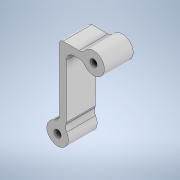
# Autodesk Inventor part: back
Saved by Autodesk Inventor 2021 (Build 250183000, 183)
## iProperties
Created: 2025-12-28
Part Number: back
Material: Generic
Document SubType Name: Modeling
Designer: Toby
Density: 1 g/cm^3
Appearance: Default
Author: Toby
Autodesk Inventor part; units mm, degrees
ref_plane "YZ Plane" through (0, 0, 0) normal (1, 0, 0) x (0, 1, 0)
ref_plane "XZ Plane" through (0, 0, 0) normal (0, 1, 0) x (-1, 0, 0)
ref_plane "XY Plane" through (0, 0, 0) normal (0, 0, 1) x (1, 0, 0)
sketch "Sketch1" plane through (0, 0, 0) normal (0, 0, 1) x (1, 0, 0)
  circle A0 centre (-5, -11) radius 3
  circle A1 centre (5, 11) radius 3
  point P0 (0, 0)
  dimension "d0" = 10
  dimension "d1" = 22
  dimension "d2" = 5
  dimension "d3" = 11
  dimension "d4" = 6
  dimension "d5" = 6
  constraints: 2 centre point, 2 coincident
  measures "d0" horizontal distance of point (-5, -11) point (5, 11)
  measures "d1" vertical distance of point (-5, -11) point (5, 11)
  measures "d2" horizontal distance of point (0, 0) point (-5, -11)
  measures "d3" vertical distance of point (-5, -11) point (0, 0)
  measures "d4" diameter of A0
  measures "d5" diameter of A1
extrude "Extrusion1" add sketch "Sketch1" along normal blind 8
sketch "Sketch2" plane through (5, 11, 8) normal (0, 0, 1) x (1, 0, 0)
  circle A0 centre (0, 0) radius 3 projected
  circle A1 centre (-10, -22) radius 3 projected
  line L0 (-10, -22) -> (-8.5, -18) construction
  line L1 (-9.0637, -22.3511) -> (-7.5637, -18.3511)
  line L2 (-9.4363, -17.6489) -> (-10.9363, -21.6489)
  arc A2 (-10.9363, -21.6489) -> (-9.0637, -22.3511) centre (-10, -22) ccw
  arc A3 (-7.5637, -18.3511) -> (-9.4363, -17.6489) centre (-8.5, -18) ccw
  circle A4 centre (-8.5, 0) radius 1
  point P0 (-5, -11)
  point P1 (-10, -19)
  point P2 (-9.25, -20)
  dimension "d8" = 0
  dimension "d9" = 1.5
  dimension "d10" = 3
  dimension "d11" = 0
  dimension "d12" = 1.5
  dimension "d13" = 4
  dimension "d14" = 2
  dimension "d15" = 2
  constraints: 8 end point, 4 point on circle, 4 tangent, 3 centre point, 1 coincident, 1 midpoint, 1 parallel
  measures "d8" vertical distance of A0.centre point (-8.5, 0)
  measures "d9" horizontal distance of L0.start point (-8.5, 0)
  measures "d10" distance of L0.start point (-10, -19)
  measures "d11" horizontal distance of L0.start point (-10, -19)
  measures "d12" horizontal distance of L0.start L0.end
  measures "d13" vertical distance of L0.start L0.end
  measures "d14" diameter of A3
  measures "d15" diameter of A4
extrude "Extrusion2" add sketch "Sketch2" against normal blind 8 contours L1 A2 L2 A1 | A1 L2 A3 L1 | A4 picked at (-9.757, -21.03)
sketch "Sketch3" plane through (-3.5, 11, 8) normal (0, 0, 1) x (1, 0, 0)
  circle A0 centre (0, 0) radius 1 projected
  circle A1 centre (8.5, 0) radius 3 projected
  line L0 (0, 0) -> (8.5, 0) construction
  line L1 (0, -1) -> (8.5, -1)
  line L2 (8.5, 1) -> (0, 1)
  arc A2 (0, 1) -> (0, -1) centre (0, 0) ccw
  arc A3 (8.5, -1) -> (8.5, 1) centre (8.5, 0) ccw
  arc A4 (0.9363, -18.3511) -> (-0.9363, -17.6489) centre (0, -18) ccw projected
  line L3 (0, 0) -> (0, -18) construction
  line L4 (-1, 0) -> (-1, -18)
  line L5 (1, -18) -> (1, 0)
  arc A5 (1, 0) -> (-1, 0) centre (0, 0) ccw
  arc A6 (-1, -18) -> (1, -18) centre (0, -18) ccw
  point P0 (3.5, -11)
  point P1 (4.25, 0)
  point P2 (0, -9)
  point P3 (1, -1)
  point P4 (-1, 0)
  constraints: 16 end point, 8 point on circle, 8 tangent, 4 centre point, 2 midpoint, 2 parallel, 1 horizontal, 1 perpendicular
extrude "Extrusion3" add sketch "Sketch3" against normal blind 8 contours A0 | L5 L1 A0 | A0 L2 A1 L1 L5 | L1 L5 A4 A6 L4 A0 | L2 A3 L1 A1 picked at (7.5064, 0.113)
fillet "Fillet1" radius 2 1 edges at (-2.5, 10, 4)
fillet "Fillet2" radius 2 4 edges at (2.1716, 10, 4) (-4.9432, -8.0005, 4) (-3.0705, -8.7028, 4) (2.1716, 12, 4)
sketch "Sketch4" plane through (0, 0, 0) normal (0, 0, -1) x (-1, 0, 0)
  arc A0 (-2.6, 12.8) -> (-2.6, 9.2) centre (-5, 11) ccw projected
  arc A1 (2.4719, -9.3848) -> (5.8427, -8.1208) centre (5, -11) ccw projected
  point P0 (0, 0)
  constraints: 2 coincident
hole "Hole1" at (5, 11, 0) at (-5, -11, 0) direction (0, 0, 1) diameter 2 depth 5 tip angle 118
sketch "Sketch5" plane through (0, 0, 8) normal (0, 0, 1) x (1, 0, 0)
  circle A0 centre (5, 11) radius 1 projected
  circle A1 centre (-5, -11) radius 1 projected
  point P0 (0, 0)
  constraints: 2 coincident
hole "Hole2" at (5, 11, 8) at (-5, -11, 8) direction (0, 0, -1) diameter 2 depth 5 tip angle 118
body "Solid1"
